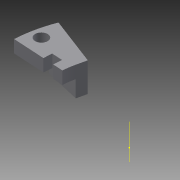
# Autodesk Inventor part: male bayonet connector 10
Saved by Autodesk Inventor 2015 (Build 190159000, 159)
## iProperties
Created: 2014-06-11
Part Number: male bayonet connector 10
Material: Generic
Document SubType Name: Modeling
Designer: ericd_000
Density: 1 g/cm^3
Appearance: Default
Author: ericd_000
Autodesk Inventor part; units mm, degrees
ref_plane "YZ Plane" through (0, 0, 0) normal (1, 0, 0) x (0, 1, 0)
ref_plane "XZ Plane" through (0, 0, 0) normal (0, 1, 0) x (-1, 0, 0)
ref_plane "XY Plane" through (0, 0, 0) normal (0, 0, 1) x (1, 0, 0)
sketch "Sketch19" plane through (0, 0, 0) normal (0, 0, 1) x (1, 0, 0)
  circle A0 centre (0, 0) radius 59
  dimension "d94" = 118
  constraints: 1 centre point, 1 coincident
  measures "d94" diameter of A0
extrude "Extrusion20" add sketch "Sketch19" along normal blind 5
sketch "Sketch21" plane through (0, 0, 5) normal (0, 0, 1) x (1, 0, 0)
  point P0 (0, 0)
sketch "Sketch23" plane through (0, 0, 5) normal (0, 0, 1) x (1, 0, 0)
  line L0 (0, 0) -> (30.298, 50.6264) construction
  circle A0 centre (0, 0) radius 59 construction
  line L1 (0, 0) -> (37.049, 45.917) construction
  circle A1 centre (0, 0) radius 59 construction
  line L2 (37.049, 45.917) -> (21.7185, 26.917)
  line L3 (21.7185, 26.917) -> (17.5881, 29.3889)
  line L4 (17.5881, 29.3889) -> (30.298, 50.6264)
  arc A2 (37.049, 45.917) -> (30.298, 50.6264) centre (0, 0) ccw
  dimension "d105" = 172
  dimension "d106" = 19
  constraints: 10 end point, 2 collinear, 2 point on circle, 1 centre point, 1 perpendicular, 5 other
  measures "d105" angle of L0 L1
  measures "d106" vertical distance of L1.end L2.end
extrude "Extrusion21" add sketch "Sketch23" along normal blind 14
sketch "Sketch26" plane through (17.5881, 29.3889, 5) normal (-0.8580744, 0.5135254, 0) x (0, 0, 1)
  line L0 (14, 24.7502) -> (14, 0)
  line L1 (14, 24.7502) -> (8, 24.7502)
  line L2 (0, 24.7502) -> (14, 24.7502) projected
  line L3 (0, 0) -> (14, 0) projected
  line L4 (8, 0) -> (14, 0)
  line L5 (8, 24.7502) -> (8, 0)
  line L6 (-8.8, -34.2498) -> (17.8, -34.2498) projected
  point P0 (-5, -34.2498)
  dimension "d122" = 6
  dimension "d123" = 6
  constraints: 8 end point, 2 point on line, 1 collinear, 1 vertical
  measures "d122" distance of L0.start L1.end
  measures "d123" distance of L4.start L0.end
revolve "Revolution2" add sketch "Sketch26" angle 9.5 about axis through (0, 0, 5) along (0, 0, 1)
sketch "Sketch25" plane through (0, 0, 19) normal (0, 0, 1) x (1, 0, 0)
  circle A0 centre (26.4944, 47.0536) radius 3
  line L0 (26.4944, 47.0536) -> (0, 0) construction
  line L1 (12.4964, 31.8887) -> (21.5267, 54.9327) projected
  dimension "d112" = 6
  dimension "d116" = 54
  dimension "d125" = 7.5
  constraints: 2 end point, 1 centre point
  measures "d112" diameter of A0
  measures "d116" distance of L0.start L0.end
  measures "d125" distance from line of L0.start L1
extrude "Extrusion22" cut sketch "Sketch25" against normal through all
sketch "Sketch27" plane through (0, 0, 19) normal (0, 0, 1) x (1, 0, 0)
  line L0 (17.5881, 29.3889) -> (21.7185, 26.917) projected
  line L1 (17.5881, 29.3889) -> (12.4964, 31.8887)
  line L2 (12.4964, 31.8887) -> (18.1594, 46.34)
  line L3 (12.4964, 31.8887) -> (21.5267, 54.9327) projected
  line L4 (18.1594, 46.34) -> (15.5726, 30.3784)
  point P0 (0, 0)
  constraints: 7 end point, 2 point on line
extrude "Extrusion23" cut sketch "Sketch27" against normal blind 10
pattern_circular "Circular Pattern2" count 10 over 360 about axis through (0, 0, 5) along (0, 0, 1) of "Extrusion21", "Revolution2", "Extrusion22", "Extrusion23"
sketch "Sketch28" plane through (0, 0, 19) normal (0, 0, 1) x (0.9776038, -0.2104537, 0)
  line L0 (-46.0823, -7.0927) -> (-33.8512, -5.2102)
  arc A0 (-34.2469, 0.4483) -> (-33.8512, -5.2102) centre (0, 0) ccw
  arc A1 (-58.3133, 8.9753) -> (-58.3133, -8.9753) centre (0, 0) ccw projected
  line L1 (-49.1918, -7.5713) -> (-58.3133, -8.9753) projected
  line L2 (-49.1918, -7.5713) -> (-34.2469, 0.4483)
  line L3 (-46.0823, -7.0927) -> (-49.1918, -7.5713)
  constraints: 6 end point, 2 collinear, 2 point on circle, 1 centre point, 1 concentric
extrude "Extrusion25" add sketch "Sketch28" against normal blind 6
sketch "Sketch29" plane through (0, 0, 5) normal (0, 0, 1) x (1, 0, 0)
  circle A0 centre (0, 0) radius 59
  line L0 (0, 0) -> (-55.1185, 21.0465)
  line L1 (0, 0) -> (-57.5112, 13.1707)
  line L2 (-55.1901, 12.6391) -> (-57.5112, 13.1707) projected
  arc A1 (-30.298, -50.6264) -> (-2.9839, -58.9245) centre (0, 0) ccw projected
  dimension "d135" = 118
  constraints: 4 end point, 1 centre point, 1 coincident, 1 collinear, 1 concentric
  measures "d135" diameter of A0
extrude "Extrusion26" cut sketch "Sketch29" against normal blind 6
sketch "Sketch30" plane through (0, 0, 5) normal (0, 0, -1) x (-1, 0, 0)
  line L0 (-109.7485, 105.489) -> (97.8298, 105.489)
  line L1 (97.8298, 105.489) -> (97.8298, -69.3705)
  line L2 (97.8298, -69.3705) -> (-109.7485, -69.3705)
  line L3 (-109.7485, -69.3705) -> (-109.7485, 105.489)
  line L4 (32.0383, -2.0031) -> (28.8173, 14.5454)
  line L5 (28.8173, 14.5454) -> (71.7406, 33.7946)
  line L6 (71.7406, 33.7946) -> (71.7406, -3.6949)
  line L7 (71.7406, -3.6949) -> (32.0383, -2.0031)
  point P0 (0, 0)
  constraints: 16 end point, 2 parallel, 1 horizontal, 1 perpendicular, 1 vertical
extrude "Extrusion27" cut sketch "Sketch30" against normal blind 16
sketch "Sketch31" plane through (-58.8962, 3.498, 19) normal (0, 0, 1) x (0.9982409, -0.0592879, 0)
  line L0 (15, 0) -> (20, 0)
  line L1 (20, 0) -> (20, 4)
  line L2 (20, 4) -> (15, 4)
  line L3 (15, 4) -> (15, 0)
  line L4 (24.7502, 0) -> (0, 0) projected
  point P0 (59, 0)
  dimension "d148" = 15
  dimension "d149" = 5
  dimension "d150" = 4
  constraints: 8 end point, 2 parallel, 1 collinear, 1 horizontal, 1 perpendicular
  measures "d148" distance from line of L3 L4.end
  measures "d149" distance of L1.end L2.end
  measures "d150" distance of L0.end L1.end
extrude "Extrusion28" cut sketch "Sketch31" against normal up to surface (6 mm away)
body "Solid2"
